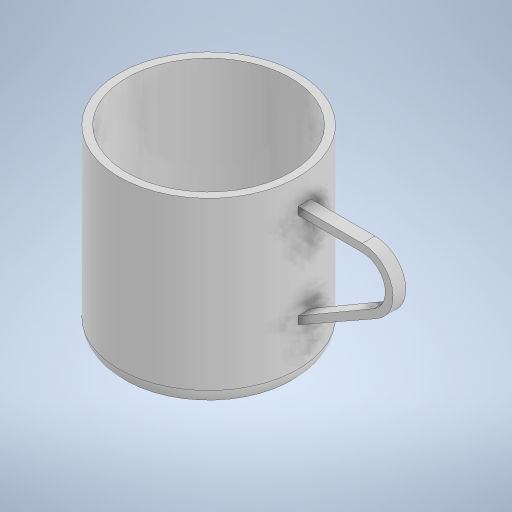
# Autodesk Inventor part: Actividad 2 Lab Dinámica Alison Martínez
Saved by Autodesk Inventor 2024 (Build 280153000, 153)
## iProperties
Created: 2024-02-25
Part Number: Actividad 2 Lab Dinámica Alison Martínez
Material: Genérico
Document SubType Name: Modeling
Designer: Alison
Density: 1 g/cm^3
Appearance: Valor por defecto
Author: Alison
Autodesk Inventor part; units mm, degrees
ref_plane "XZ Plane" through (0, 0, 0) normal (0, 1, 0) x (-1, 0, 0)
sketch "Boceto1" plane through (0, 0, 0) normal (0, 0, 1) x (1, 0, 0)
  line L0 (0, 0) -> (0, 70)
  line L1 (0, 70) -> (-35, 70)
  line L2 (-35, 70) -> (-35, 5)
  line L3 (0, 0) -> (-32.5, 0)
  arc A0 (-35, 5) -> (-32.5, 0) centre (-28.75, 5) ccw
  constraints: 8 end point, 2 horizontal, 2 point on circle, 1 centre point, 1 perpendicular, 1 tangent, 1 vertical
revolve "Revolución1" add sketch "Boceto1" angle 360 about axis through (0, 0, 0) along (0, 1, 0)
shell "Vaciado2" thickness 3 removed faces 1 at (-0.2748, 70, -9.3581)
sketch "Boceto2" plane through (0, 0, 0) normal (0, 0, 1) x (1, 0, 0)
  line L0 (35, 5) -> (35, 70) projected
  line L1 (35, 70) -> (35, 60)
  line L2 (35, 60) -> (60, 60)
  line L3 (35, 5) -> (35, 20)
  arc A0 (65.9265, 37.5656) -> (60, 60) centre (60, 48) ccw
  line L4 (35, 20) -> (65.9265, 37.5656)
  line L5 (35, 60) -> (35, 57)
  line L6 (35, 60) -> (35, 57)
  line L7 (35, 57) -> (60, 57)
  arc A1 (65.2003, 40.6545) -> (60, 57) centre (60, 48) ccw
  line L8 (35, 20) -> (35, 23)
  line L9 (35, 5) -> (35, 70) projected
  line L10 (35, 23) -> (65.2003, 40.6545)
  point P0 (0, 0)
  dimension "d11" = 10
  dimension "d12" = 25
  dimension "d13" = 15
  dimension "d20" = 12
  dimension "d23" = 3
  dimension "d24" = 3
  dimension "d26" = 3
  constraints: 18 end point, 4 point on circle, 4 point on line, 3 tangent, 2 centre point, 2 perpendicular, 1 collinear, 1 concentric
  measures "d11" distance of L0.end L1.end
  measures "d12" distance of L1.end L2.end
  measures "d13" distance of L0.start L3.end
  measures "d20" radius of A0
  measures "d23" distance of L1.end L5.end
  measures "d24" distance of L1.end L5.end
  measures "d26" distance of L3.end L8.end
ref_plane "Plano de trabajo7" through (60, 60, 0) normal (0, 0, 1) x (1, 0, 0)
ref_plane "Plano de trabajo8" through (35, 60, 0) normal (1, 0, 0) x (0, 1, 0)
extrude "Extrusión1" add sketch "Boceto2" against normal blind 5
sketch "Boceto5" plane through (0, 0, -5) normal (0, 0, -1) x (-1, 0, 0)
  point P0 (0, 0)
sketch "Boceto6" plane through (0, 0, -5) normal (0, 0, -1) x (-1, 0, 0)
  line L0 (-35, 20) -> (-35, 60) projected
  line L1 (-35, 20) -> (-35, 23)
  line L2 (-35, 60) -> (-60, 60) projected
  line L3 (-35, 60) -> (-35, 57)
  line L4 (-35, 57) -> (-60, 57)
  arc A0 (-60, 57) -> (-63.3814, 39.6594) centre (-60, 48) ccw
  arc A1 (-63.3814, 39.6594) -> (-64.5343, 40.2257) centre (-60, 48) ccw
  line L5 (-35, 23) -> (-64.5343, 40.2257)
  line L6 (-35, 57) -> (-35, 23)
  point P0 (0, 0)
  dimension "d27" = 3
  dimension "d28" = 3
  dimension "d29" = 25
  dimension "d30" = 9
  constraints: 10 end point, 5 point on circle, 4 tangent, 2 centre point, 2 point on line, 1 collinear, 1 concentric, 1 perpendicular
  measures "d27" distance of L0.start L1.end
  measures "d28" distance of L0.end L3.end
  measures "d29" distance of L3.end L4.end
  measures "d30" radius of A0
extrude "Extrusión2" cut sketch "Boceto6" against normal blind 5
